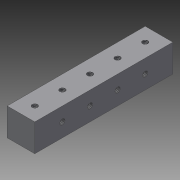
# Autodesk Inventor part: Lead_Screw_Fixture_Side_Wall
Saved by Autodesk Inventor 2015 (Build 190159000, 159)
## iProperties
Created: 2014-12-22
Part Number: Lead_Screw_Fixture_Side_Wall
Material: Generic
Document SubType Name: Modeling
Designer: Drew
Density: 1 g/cm^3
Appearance: Default
Author: Drew
Autodesk Inventor part; units mm, degrees
ref_plane "YZ Plane" through (0, 0, 0) normal (1, 0, 0) x (0, 1, 0)
ref_plane "XZ Plane" through (0, 0, 0) normal (0, 1, 0) x (-1, 0, 0)
ref_plane "XY Plane" through (0, 0, 0) normal (0, 0, 1) x (1, 0, 0)
sketch "Sketch1" plane through (0, 0, 0) normal (0, 1, 0) x (-1, 0, 0)
  line L0 (-6.35, -31.75) -> (6.35, -31.75)
  line L1 (6.35, -31.75) -> (6.35, 31.75)
  line L2 (6.35, 31.75) -> (-6.35, 31.75)
  line L3 (-6.35, 31.75) -> (-6.35, -31.75)
  line L4 (-6.35, -31.75) -> (6.35, 31.75) construction
  line L5 (6.35, -31.75) -> (-6.35, 31.75) construction
  point P0 (0, 0)
  dimension "d0" = 63.5
  dimension "d1" = 12.7
  constraints: 12 end point, 2 midpoint, 2 parallel, 1 horizontal, 1 perpendicular
  measures "d0" distance of L0.end L1.end
  measures "d1" distance of L1.end L2.end
extrude "Extrusion1" add sketch "Sketch1" along normal blind 12.7
sketch "Sketch2" plane through (6.35, 0, 31.75) normal (1, 0, 0) x (0, 0, -1)
  line L0 (63.5, 0) -> (63.5, 12.7) projected
  line L1 (63.5, 6.35) -> (0, 6.35)
  line L2 (0, 0) -> (0, 12.7) projected
  line L3 (31.75, 6.35) -> (31.75, 12.7)
  point P0 (31.75, 0)
  point P1 (12.7, 6.35)
  point P2 (25.4, 6.35)
  point P3 (38.1, 6.35)
  point P4 (50.8, 6.35)
  dimension "d4" = 12.7
  dimension "d5" = 12.7
  dimension "d6" = 12.7
  dimension "d15" = 6.35
  constraints: 4 end point, 4 point on line, 3 midpoint, 1 vertical
  measures "d4" distance of point (25.4, 6.35) point (12.7, 6.35)
  measures "d5" distance of point (38.1, 6.35) point (25.4, 6.35)
  measures "d6" distance of point (50.8, 6.35) point (38.1, 6.35)
  measures "d15" distance from line of point (25.4, 6.35) L3
hole "Hole1" at (6.35, 6.35, 19.05) at (6.35, 6.35, 6.35) at (6.35, 6.35, -6.35) at (6.35, 6.35, -19.05) direction (-1, 0, 0) diameter 2.4638 end through all
sketch "Sketch3" plane through (0, 0, 0) normal (0, -1, 0) x (1, 0, 0)
  line L0 (6.35, 31.75) -> (6.35, -31.75) projected
  line L1 (6.35, 0) -> (-6.35, 0)
  line L2 (-6.35, -31.75) -> (-6.35, 31.75) projected
  point P0 (0, 0)
  point P1 (0, 25.4)
  point P2 (0, 12.7)
  point P3 (0, -12.7)
  point P4 (0, -25.4)
  point P5 (0, 0)
  dimension "d16" = 12.7
  dimension "d17" = 12.7
  dimension "d18" = 12.7
  dimension "d19" = 12.7
  constraints: 2 end point, 2 midpoint, 1 coincident
  measures "d16" distance of point (0, 12.7) point (0, 25.4)
  measures "d17" distance of point (0, 0) point (0, 12.7)
  measures "d18" distance of point (0, -12.7) point (0, 0)
  measures "d19" distance of point (0, -25.4) point (0, -12.7)
hole "Hole2" at (0, 0, 25.4) at (0, 0, 12.7) at (0, 0, -12.7) at (0, 0, -25.4) at (0, 0, 0) direction (0, 1, 0) diameter 2.4638 end through all
equation "\"d5\" = d4"
equation "\"d6\" = d5"
equation "\"d15\" = 0.5 * d5"
equation "\"d17\" = d16"
equation "\"d18\" = d17"
equation "\"d19\" = d18"
body "Solid1"
